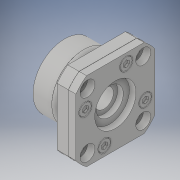
# Autodesk Inventor part: C-TFK10_b
Saved by Autodesk Inventor 2019 (Build 230136000, 136)
## iProperties
Created: 2023-03-01
Part Number: C-TFK10_b
Material: Generic
Catalog Web Link: www.cadenas.de
Description: C-TFK_b-Economy Support Units Fixed Side Round
Vendor: MISUMI
Document SubType Name: Modeling
Designer: psAdmin
Manufacturer: MISUMI
Mass: 26.9127 g
Surface Area: 85.783 cm^2
Volume: 26.9127 cm^3
Density: 1 g/cm^3
Appearance: PSOLRGB-175-175-175
Category: PARTsolutions
Company: MISUMI
Title: C-TFK10
Author: Cadenas PARTsolutions
Comments: Economy Support Units Fixed Side Round
PSOL_IDENT_0: {$CADENAS_DATA/23d-libs/misumi/metric/09_ball_screws/c_tfk/c_tfk_base.prj},161 {VTYP=3D},{NB=C-TFK10
PSOL_IDENT_1: _b},{LINA=C-TFK10},{NN=C-TFK_b},{DATE=14.09.2022 01:47:56},{GEOMDATE=16.11.2021 00:37:14},{VERSION=}
PSOL_IDENT_2: ,{LINEID=100},{WBVAR=SET},{WBNUMERIC=}  {NB=C-TFK10_b},{LINA=C-TFK10},{KT=DUMMY},{PN=C-TFK10},{TYPE=
PSOL_IDENT_3: C-TFK},{NO=10},{SET=},{DD=10},{L=27},{H=10},{F=17},{E=29.5},{D=34},{A=52},{PCD=42},{B=42},{L1=7.5},{
PSOL_IDENT_4: T1=5.0},{DD1=4.5},{DD2=8.0},{LL=4.0},{M=M10x1.0},{T=16},{ACD=14.5},{ACV=10},{ACL=5.5},{SID=14.0},{Z1=
PSOL_IDENT_5: 22},{Z2=14.5},{Z3=6.0},{Z4=3.0},{Z5=21},{X1=7},{X2=6.2},{X3=3.00},{X4=34},{CP=10},{Y1=0},{Y2=0.0},{Y
PSOL_IDENT_6: 3=0.0},{Y4=0},{B1=2.3},{B2=4.55},{NO2=10},{ACNM=M10x1.0},{ACNB=8.0},{ACNMM=M3},{ACNDD=15},{ACND=20.0
PSOL_IDENT_7: },{ACNF=16}
NB: C-TFK10_b
NN: C-TFK_b
NT: Economy Support Units Fixed Side Round
NBSYN: $PN._b
LINA: C-TFK10
CATALOG: Misumi
PN: C-TFK10
NO: 10
SET: w/o SET
DD: 10
L: 27
H: 10
F: 17
E: 29.5
D: 34
A: 52
PCD: 42
B: 42
L1: 7.5
T1: 5
DD1: 4.5
DD2: 8
LL: 4
M: M10x1.0
T: 16
ACD: 14.5
ACV: 10
ACL: 5.5
ACNM: M10x1.0
ACNB: 8
ACNMM: M3
ACNDD: 15
ACND: 20
ACNF: 16
SUPPLIER: MISUMI
ARTICLENO: C-TFK10_b
BOMINFO: C-TFK10
CREATOR: CADENAS GmbH
Autodesk Inventor part; units mm, degrees
ref_plane "YZ Plane" through (0, 0, 0) normal (1, 0, 0) x (0, 1, 0)
ref_plane "XZ Plane" through (0, 0, 0) normal (0, 1, 0) x (-1, 0, 0)
ref_plane "XY Plane" through (0, 0, 0) normal (0, 0, 1) x (1, 0, 0)
sketch "Sketch_1" plane through (0, 0, 0) normal (0, 0, 1) x (1, 0, 0)
  line L0 (17, 0) -> (0, 0)
  line L1 (0, 0) -> (0, 17)
  line L2 (0, 17) -> (16.7, 17)
  arc A0 (16.7, 17) -> (17, 17.3) centre (16.7, 17.3) ccw
  line L3 (17, 17.3) -> (17, 0)
  line L4 (17, 0) -> (0, 0)
  constraints: 10 end point, 2 point on circle, 1 centre point
revolve "Revolution1" add sketch "Sketch_1" angle 360 about axis through (17, 0, 0) along (1, 0, 0)
sketch "Sketch_2" plane through (17, 0, 0) normal (1, 0, 0) x (0, 0, -1)
  line L0 (-21, 15.3297) -> (-21, -15.3297)
  arc A0 (-21, -15.3297) -> (-15.3297, -21) centre (0, 0) ccw
  line L1 (-15.3297, -21) -> (15.3297, -21)
  arc A1 (15.3297, -21) -> (21, -15.3297) centre (0, 0) ccw
  line L2 (21, -15.3297) -> (21, 15.3297)
  arc A2 (21, 15.3297) -> (15.3297, 21) centre (0, 0) ccw
  line L3 (15.3297, 21) -> (-15.3297, 21)
  arc A3 (-15.3297, 21) -> (-21, 15.3297) centre (0, 0) ccw
  constraints: 8 end point, 8 point on circle, 4 centre point
extrude "Extrusion1" add sketch "Sketch_2" along normal blind 10
sketch "_____4" plane through (0, 0, 0) normal (0, 0, 1) x (1, 0, 0)
  line L0 (54, 0) -> (-54, 0)
  line L1 (14.7, 17) -> (15, 16.7)
  line L2 (15, 16.7) -> (16.8, 16.7)
  arc A0 (16.8, 16.7) -> (17.3, 17.2) centre (16.8, 17.2) ccw
  line L3 (17.3, 17.2) -> (17.3, 19)
  line L4 (17.3, 19) -> (17, 19.3)
  line L5 (17, 19.3) -> (14.7, 17)
  constraints: 12 end point, 2 point on circle, 1 centre point
revolve "Revolution2" cut sketch "_____4" angle 360 about axis through (54, 0, 0) along (1, 0, 0)
sketch "_____5" plane through (0, 0, 0) normal (0, 0, 1) x (1, 0, 0)
  line L0 (54, 0) -> (-54, 0)
  line L1 (0, 17) -> (0, 16.85)
  line L2 (0, 16.85) -> (10, 16.85)
  line L3 (10, 16.85) -> (10.15, 17)
  line L4 (10.15, 17) -> (0, 17)
  constraints: 10 end point
revolve "Revolution3" cut sketch "_____5" angle 360 about axis through (54, 0, 0) along (1, 0, 0)
sketch "Sketch_5" plane through (0, 0, 0) normal (0, 0, 1) x (1, 0, 0)
  line L0 (27, 0) -> (0, 0)
  line L1 (0, 0) -> (0, 10.5)
  line L2 (0, 10.5) -> (2, 10.5)
  line L3 (2, 10.5) -> (2, 7.25)
  line L4 (2, 7.25) -> (5, 7.25)
  line L5 (5, 7.25) -> (5, 5)
  line L6 (5, 5) -> (21, 5)
  line L7 (21, 5) -> (21, 7.25)
  line L8 (21, 7.25) -> (24, 7.25)
  line L9 (24, 7.25) -> (24, 10.5)
  line L10 (24, 10.5) -> (27, 11)
  line L11 (27, 11) -> (27, 0)
  line L12 (27, 0) -> (0, 0)
  constraints: 26 end point
revolve "Revolution4" cut sketch "Sketch_5" angle 360 about axis through (27, 0, 0) along (1, 0, 0)
sketch "Sketch6" plane through (27, 0, 0) normal (1, 0, 0) x (0, 0, -1)
  point P0 (-14.8492, -14.8492)
hole "Hole1" at (27, -14.8492, 14.8492) direction (-1, 0, 0) diameter 4.5 depth 10 counterbore diameter 8 counterbore depth 4
pattern_linear "Rectangular Pattern1" count 2 spacing 29.6985 along (0, 0, -1) count 2 spacing 29.6985 along (0, 1, 0) of "Hole1"
sketch "Sketch_9" plane through (23, 0, 0) normal (1, 0, 0) x (0, 0, -1)
  line L0 (-21, 15.3297) -> (-21, -15.3297)
  arc A0 (-21, -15.3297) -> (-15.3297, -21) centre (0, 0) ccw
  line L1 (-15.3297, -21) -> (15.3297, -21)
  arc A1 (15.3297, -21) -> (21, -15.3297) centre (0, 0) ccw
  line L2 (21, -15.3297) -> (21, 15.3297)
  arc A2 (21, 15.3297) -> (15.3297, 21) centre (0, 0) ccw
  line L3 (15.3297, 21) -> (-15.3297, 21)
  arc A3 (-15.3297, 21) -> (-21, 15.3297) centre (0, 0) ccw
  line L4 (-20.95, 15.3134) -> (-20.95, -15.3134)
  arc A4 (-20.95, -15.3134) -> (-15.3134, -20.95) centre (0, 0) ccw
  line L5 (-15.3134, -20.95) -> (15.3134, -20.95)
  arc A5 (15.3134, -20.95) -> (20.95, -15.3134) centre (0, 0) ccw
  line L6 (20.95, -15.3134) -> (20.95, 15.3134)
  arc A6 (20.95, 15.3134) -> (15.3134, 20.95) centre (0, 0) ccw
  line L7 (15.3134, 20.95) -> (-15.3134, 20.95)
  arc A7 (-15.3134, 20.95) -> (-20.95, 15.3134) centre (0, 0) ccw
  constraints: 16 end point, 16 point on circle, 8 centre point
extrude "Extrusion2" cut sketch "Sketch_9" along normal mid plane 0.05
sketch "Sketch_10" plane through (27, 0, 0) normal (1, 0, 0) x (0, 0, -1)
  circle A0 centre (-15.9748, 5.8143) radius 3.5
  circle A1 centre (-15.9748, 5.8143) radius 3.1
  constraints: 2 centre point
extrude "Extrusion3" cut sketch "Sketch_10" against normal blind 1
pattern_linear "Rectangular Pattern2" count 2 spacing 24.0416 along (0, 0.4226183, -0.9063078) count 2 spacing 24.0416 along (0, -0.9063078, -0.4226183) of "Extrusion3"
sketch "Sketch_12" plane through (27, 0, 0) normal (1, 0, 0) x (0, 0, -1)
  line L0 (-17.4748, 4.9483) -> (-15.9748, 4.0823)
  line L1 (-15.9748, 4.0823) -> (-14.4748, 4.9483)
  line L2 (-14.4748, 4.9483) -> (-14.4748, 6.6804)
  line L3 (-14.4748, 6.6804) -> (-15.9748, 7.5464)
  line L4 (-15.9748, 7.5464) -> (-17.4748, 6.6804)
  line L5 (-17.4748, 6.6804) -> (-17.4748, 4.9483)
  constraints: 12 end point
extrude "Extrusion4" cut sketch "Sketch_12" against normal blind 1
pattern_linear "Rectangular Pattern3" count 2 spacing 24.0416 along (0, 0.4226183, -0.9063078) count 2 spacing 24.0416 along (0, -0.9063078, -0.4226183) of "Extrusion4"
ref_plane "_to_bjs_XY" through (27, 0, 0) normal (1, 0, 0) x (0, 0, -1)
ref_plane "_to_bjs_YZ" through (27, 0, 0) normal (0, 0, -1) x (0, 1, 0)
ref_plane "_to_bjs_ZX" through (27, 0, 0) normal (0, 1, 0) x (1, 0, 0)
ref_plane "to_collar_XY" through (21, 0, 0) normal (-1, 0, 0) x (0, 0, -1)
ref_plane "to_collar_YZ" through (21, 0, 0) normal (0, 0, -1) x (0, -1, 0)
ref_plane "to_collar_ZX" through (21, 0, 0) normal (0, -1, 0) x (-1, 0, 0)
ref_plane "to_collar_2_XY" through (5, 0, 0) normal (1, 0, 0) x (0, 0, -1)
ref_plane "to_collar_2_YZ" through (5, 0, 0) normal (0, 0, -1) x (0, 1, 0)
ref_plane "to_collar_2_ZX" through (5, 0, 0) normal (0, 1, 0) x (1, 0, 0)
ref_plane "to_dummy_XY" through (0, 0, 0) normal (1, 0, 0) x (0, 0, -1)
ref_plane "to_dummy_YZ" through (0, 0, 0) normal (0, 0, -1) x (0, 1, 0)
ref_plane "to_dummy_ZX" through (0, 0, 0) normal (0, 1, 0) x (1, 0, 0)
body "Solid1"
